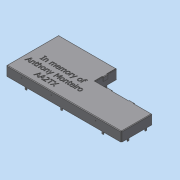
# Autodesk Inventor part: tx_v2_04_cu_shield
Saved by Autodesk Inventor 2014 (Build 180170000, 170)
## iProperties
Created: 2014-03-05
Part Number: tx_v2_04_cu_shield
Material: Generic
Document SubType Name: Sheet Metal
Designer: Robert Davis
Density: 1 g/cm^3
Sheet Metal Rule: Default_mm
Appearance: Default
Flat Pattern Width: 6.62019 cm
Flat Pattern Length: 9.2582 cm
Flat Pattern Area: 61.291 cm^2
Sheet Metal Width: 66.2019 mm
Sheet Metal Length: 92.5820 mm
Sheet Metal Area: 6129.1043 mm^2
Author: Robert Davis
Autodesk Inventor part; units mm, degrees
ref_plane "YZ Plane" through (0, 0, 0) normal (1, 0, 0) x (0, 1, 0)
ref_plane "XZ Plane" through (0, 0, 0) normal (0, 1, 0) x (-1, 0, 0)
ref_plane "XY Plane" through (0, 0, 0) normal (0, 0, 1) x (1, 0, 0)
sketch "Sketch1" plane through (0, 0, 0) normal (0, 0, 1) x (1, 0, 0)
  line L0 (7.5, 46.3001) -> (22.25, 46.3001)
  line L1 (22.25, 46.3001) -> (22.25, 52.2431)
  line L2 (-31.08, 52.2431) -> (-31.08, 45.9911)
  line L3 (-31.08, 45.9911) -> (-37.332, 45.9911)
  line L4 (-37.332, 11.4131) -> (-31.08, 11.4131)
  line L5 (-31.08, 11.4131) -> (-31.08, 5.1611)
  line L6 (45.998, 5.1611) -> (45.998, 11.4131)
  line L7 (45.998, 11.4131) -> (52.25, 11.4131)
  line L8 (52.25, 69.863) -> (46.307, 69.863)
  line L9 (46.307, 69.863) -> (46.307, 31.493)
  line L10 (-17.791, 5.1611) -> (-17.791, 3.6611)
  line L11 (-17.791, 3.6611) -> (-18.791, 3.6611)
  line L12 (-18.791, 3.6611) -> (-18.791, 5.1611)
  line L13 (6.209, 5.1611) -> (6.209, 3.6611)
  line L14 (6.209, 3.6611) -> (5.209, 3.6611)
  line L15 (5.209, 3.6611) -> (5.209, 5.1611)
  line L16 (34.209, 5.1611) -> (34.209, 3.6611)
  line L17 (34.209, 3.6611) -> (33.209, 3.6611)
  line L18 (33.209, 3.6611) -> (33.209, 5.1611)
  line L19 (-31.08, 5.1611) -> (-18.791, 5.1611)
  line L20 (34.209, 5.1611) -> (45.998, 5.1611)
  line L21 (-17.791, 5.1611) -> (5.209, 5.1611)
  line L22 (6.209, 5.1611) -> (33.209, 5.1611)
  line L23 (-37.332, 16.7021) -> (-38.832, 16.7021)
  line L24 (-38.832, 16.7021) -> (-38.832, 17.7021)
  line L25 (-38.832, 17.7021) -> (-37.332, 17.7021)
  line L26 (-37.332, 36.7021) -> (-38.832, 36.7021)
  line L27 (-38.832, 36.7021) -> (-38.832, 37.7021)
  line L28 (-38.832, 37.7021) -> (-37.332, 37.7021)
  line L29 (-18.791, 52.2431) -> (-18.791, 53.7431)
  line L30 (-18.791, 53.7431) -> (-19.791, 53.7431)
  line L31 (-19.791, 53.7431) -> (-19.791, 52.2431)
  line L32 (-3.291, 52.2431) -> (-3.291, 53.7431)
  line L33 (-3.291, 53.7431) -> (-4.291, 53.7431)
  line L34 (-4.291, 53.7431) -> (-4.291, 52.2431)
  line L35 (-4.291, 52.2431) -> (-18.791, 52.2431)
  line L36 (-19.791, 52.2431) -> (-31.08, 52.2431)
  line L37 (-37.332, 45.9911) -> (-37.332, 37.7021)
  line L38 (-37.332, 36.7021) -> (-37.332, 17.7021)
  line L39 (-37.332, 16.7021) -> (-37.332, 11.4131)
  line L40 (15.091, 52.2431) -> (15.091, 53.7431)
  line L41 (15.091, 53.7431) -> (14.091, 53.7431)
  line L42 (14.091, 53.7431) -> (14.091, 52.2431)
  line L43 (52.25, 15.2021) -> (53.75, 15.2021)
  line L44 (53.75, 15.2021) -> (53.75, 16.2021)
  line L45 (53.75, 16.2021) -> (52.25, 16.2021)
  line L46 (52.25, 27.2021) -> (53.75, 27.2021)
  line L47 (53.75, 27.2021) -> (53.75, 28.2021)
  line L48 (53.75, 28.2021) -> (52.25, 28.2021)
  line L49 (52.25, 42.5821) -> (53.75, 42.5821)
  line L50 (53.75, 42.5821) -> (53.75, 43.5821)
  line L51 (53.75, 43.5821) -> (52.25, 43.5821)
  line L52 (52.25, 60.5821) -> (53.75, 60.5821)
  line L53 (53.75, 60.5821) -> (53.75, 61.5821)
  line L54 (53.75, 61.5821) -> (52.25, 61.5821)
  line L55 (22.25, 52.2431) -> (15.091, 52.2431)
  line L56 (14.091, 52.2431) -> (-3.291, 52.2431)
  line L57 (52.25, 61.5821) -> (52.25, 69.863)
  line L58 (52.25, 43.5821) -> (52.25, 60.5821)
  line L59 (52.25, 11.4131) -> (52.25, 15.2021)
  line L60 (52.25, 16.2021) -> (52.25, 27.2021)
  line L61 (52.25, 28.2021) -> (52.25, 42.5821)
  line L62 (7.5, 39.993) -> (10.5, 39.993)
  line L63 (10.5, 39.993) -> (10.5, 36.993)
  line L64 (10.5, 36.993) -> (7.5, 36.993)
  line L65 (31, 31.493) -> (31, 34.493)
  line L66 (31, 34.493) -> (34, 34.493)
  line L67 (34, 34.493) -> (34, 31.493)
  line L68 (16, 31.493) -> (16, 34.493)
  line L69 (16, 34.493) -> (19, 34.493)
  line L70 (19, 34.493) -> (19, 31.493)
  line L71 (7.5, 31.493) -> (7.5, 36.993)
  line L72 (7.5, 39.993) -> (7.5, 46.3001)
  line L73 (34, 31.493) -> (46.307, 31.493)
  line L74 (7.5, 31.493) -> (16, 31.493)
  line L75 (19, 31.493) -> (31, 31.493)
  circle A0 centre (-21.08, 9.1611) radius 0.25
  circle A1 centre (-1.08, 9.1611) radius 0.25
  circle A2 centre (28.92, 9.1611) radius 0.25
  point P0 (0, 0)
  point P1 (-18.291, 3.6611)
  point P2 (5.709, 3.6611)
  point P3 (33.709, 3.6611)
  point P4 (-38.832, 17.2021)
  point P5 (-38.832, 37.2021)
  point P6 (-19.291, 53.7431)
  point P7 (-3.791, 53.7431)
  point P8 (14.591, 53.7431)
  point P9 (53.75, 61.0821)
  point P10 (53.75, 43.0821)
  point P11 (53.75, 27.7021)
  point P12 (53.75, 15.7021)
  point P13 (10.5, 38.493)
  point P14 (17.5, 34.493)
  point P15 (32.5, 34.493)
  dimension "d3" = 14.75
  dimension "d4" = 14.8071
  dimension "d5" = 6.252
  dimension "d7" = 34.578
  dimension "d8" = 77.078
  dimension "d9" = 38.37
  dimension "d10" = 5.943
  dimension "d60" = 5.943
  dimension "d74" = 1.5
  dimension "d75" = 1
  dimension "d76" = 12.789
  dimension "d77" = 24
  dimension "d78" = 28
  dimension "d79" = 5.789
  dimension "d80" = 20
  dimension "d81" = 11.789
  dimension "d82" = 15.5
  dimension "d83" = 4.289
  dimension "d84" = 12
  dimension "d85" = 15.38
  dimension "d86" = 18
  dimension "d87" = 18.382
  dimension "d89" = 38.58
  dimension "d90" = 7.5
  dimension "d91" = 31.493
  dimension "d92" = 3
  dimension "d93" = 3
  dimension "d94" = 7
  dimension "d95" = 10
  dimension "d96" = 15
  dimension "d117" = 0.5
  dimension "d118" = 20
  dimension "d119" = 30
  dimension "d120" = 10
  dimension "d121" = 4
  constraints: 152 end point, 46 equal length, 31 horizontal, 23 vertical, 15 midpoint, 15 parallel, 7 perpendicular, 3 centre point, 2 equal radius
  measures "d3" distance of L0.start L0.end
  measures "d4" distance of L71.start L0.start
  measures "d5" distance of L2.start L2.end
  measures "d7" distance of L3.end L4.start
  measures "d8" distance of L5.end L6.start
  measures "d9" distance of L8.end L9.end
  measures "d10" distance of L0.end L1.end
  measures "d60" distance of L8.start L8.end
  measures "d74" distance of L11.end L12.end
  measures "d75" distance of L10.end L11.end
  measures "d76" distance from line of point (-18.291, 3.661) L5
  measures "d77" distance of point (5.709, 3.661) point (-18.291, 3.661)
  measures "d78" distance of point (33.709, 3.661) point (5.709, 3.661)
  measures "d79" distance from line of point (-38.832, 17.202) L4
  measures "d80" distance of point (-38.832, 37.202) point (-38.832, 17.202)
  measures "d81" distance from line of point (-19.291, 53.743) L2
  measures "d82" distance of point (-3.791, 53.743) point (-19.291, 53.743)
  measures "d83" distance from line of point (53.75, 15.702) L7
  measures "d84" distance of point (53.75, 27.702) point (53.75, 15.702)
  measures "d85" distance of point (53.75, 43.082) point (53.75, 27.702)
  measures "d86" distance of point (53.75, 61.082) point (53.75, 43.082)
  measures "d87" distance of point (14.591, 53.743) point (-3.791, 53.743)
  measures "d89" distance between parallel lines of L2 L72
  measures "d90" distance from line of point (0, 0) L71
  measures "d91" distance from line of point (0, 0) L74
  measures "d92" distance of L62.end L63.end
  measures "d93" distance of L62.start L62.end
  measures "d94" distance from line of point (10.5, 38.493) L74
  measures "d95" distance from line of point (17.5, 34.493) L71
  measures "d96" distance of point (32.5, 34.493) point (17.5, 34.493)
  measures "d117" diameter of A0
  measures "d118" distance of A1.centre A0.centre
  measures "d119" distance of A2.centre A1.centre
  measures "d120" distance from line of A0.centre L5
  measures "d121" distance from line of A0.centre L19
extrude "Plate1" add sketch "Sketch1" along normal blind 0.381
sketch "Sketch4" plane through (0, 0, 0) normal (0, 0, -1) x (-1, 0, 0)
  line L0 (-7.5, 31.493) -> (-7.5, 46.3001) projected
  line L1 (31.08, 52.2431) -> (31.08, 45.9911) projected
  line L2 (31.08, 46.1431) -> (-7.5, 46.1431)
  line L3 (-22.25, 52.2431) -> (31.08, 52.2431) projected
  point P0 (0, 0)
  dimension "d61" = 6.1
  constraints: 2 end point, 2 point on line, 1 horizontal
  measures "d61" distance between parallel lines of L3 L2
fold "Fold2" angle 90 bend radius 0.001 thickness 0.381 k factor 0.44 line from (-31.08, 46.1431, 0) to (7.5, 46.1431, 0) line at bend centre moving side (0, 1, 0) folds toward (0, 0, -1)
sketch "Sketch5" plane through (-31.08, 46.0117, -5.9686) normal (0, -1, 0) x (1, 0, 0)
  line L0 (53.33, 0) -> (0, 0) projected
  line L1 (38.58, 5.943) -> (53.33, 5.943) projected
  line L2 (38.73, 5.943) -> (38.73, 0)
  line L3 (53.33, 5.943) -> (53.33, 0) projected
  point P0 (31.08, 5.9686)
  dimension "d62" = 14.6
  constraints: 2 end point, 2 point on line, 1 vertical
  measures "d62" distance between parallel lines of L2 L3
fold "Fold3" angle 90 bend radius 0.001 thickness 0.381 k factor 0.44 line from (7.65, 46.0117, -0.0256) to (7.65, 46.0117, -5.9686) line at bend centre moving side (1, 0, 0) folds toward (0, -1, 0)
sketch "Sketch6" plane through (0, 0, 0) normal (0, 0, -1) x (-1, 0, 0)
  line L0 (37.332, 11.4131) -> (31.08, 11.4131) projected
  line L1 (31.08, 45.9911) -> (37.332, 45.9911) projected
  line L2 (31.232, 45.9911) -> (31.232, 11.4131)
  line L3 (37.332, 45.9911) -> (37.332, 11.4131) projected
  point P0 (0, 0)
  dimension "d63" = 6.1
  constraints: 2 end point, 2 point on line, 1 vertical
  measures "d63" distance between parallel lines of L3 L2
fold "Fold4" angle 90 bend radius 0.001 thickness 0.381 k factor 0.44 line from (-31.232, 45.9911, 0) to (-31.232, 11.4131, 0) line at bend centre moving side (-1, 0, 0) folds toward (0, 0, -1)
sketch "Sketch7" plane through (0, 0, 0) normal (0, 0, -1) x (-1, 0, 0)
  line L0 (-45.998, 5.1611) -> (-45.998, 11.4131) projected
  line L1 (31.08, 11.4131) -> (31.08, 5.1611) projected
  line L2 (-45.998, 11.2611) -> (31.08, 11.2611)
  line L3 (31.08, 5.1611) -> (-45.998, 5.1611) projected
  point P0 (0, 0)
  dimension "d64" = 6.1
  constraints: 2 end point, 2 point on line, 1 horizontal
  measures "d64" distance between parallel lines of L3 L2
fold "Fold5" angle 90 bend radius 0.001 thickness 0.381 k factor 0.44 line from (45.998, 11.2611, 0) to (-31.08, 11.2611, 0) line at bend centre moving side (0, -1, 0) folds toward (0, 0, -1)
sketch "Sketch8" plane through (0, 0, 0) normal (0, 0, -1) x (-1, 0, 0)
  line L0 (-46.307, 31.493) -> (-7.5, 31.493) projected
  line L1 (-45.998, 11.4131) -> (-52.25, 11.4131) projected
  line L2 (-46.15, 11.4131) -> (-46.15, 31.493)
  line L3 (-52.25, 11.4131) -> (-52.25, 69.863) projected
  point P0 (0, 0)
  dimension "d65" = 6.1
  constraints: 2 end point, 2 point on line, 1 vertical
  measures "d65" distance between parallel lines of L2 L3
fold "Fold6" angle 90 bend radius 0.001 thickness 0.381 k factor 0.44 line from (46.15, 11.4131, 0) to (46.15, 31.493, 0) line at bend centre moving side (1, 0, 0) folds toward (0, 0, -1)
sketch "Sketch9" plane through (46.0186, 11.4131, -5.9686) normal (-1, 0, 0) x (0, 0, 1)
  line L0 (5.943, 58.4499) -> (5.943, 20.0799) projected
  line L1 (0, 0) -> (0, 58.4499) projected
  line L2 (5.943, 20.2299) -> (0, 20.2299)
  line L3 (0, 58.4499) -> (5.943, 58.4499) projected
  point P0 (5.9686, -11.4131)
  dimension "d66" = 38.22
  constraints: 2 end point, 2 point on line, 1 horizontal
  measures "d66" distance between parallel lines of L3 L2
fold "Fold7" angle 90 bend radius 0.001 thickness 0.381 k factor 0.44 line from (46.0186, 31.643, -0.0256) to (46.0186, 31.643, -5.9686) line at bend centre moving side (0, 1, 0) folds toward (-1, 0, 0)
ref_plane "Work Plane1" through (-31.08, 11.202, -5.9686) normal (0, 1, 0) x (1, 0, 0)
ref_plane "Work Plane2" through (-31.2911, 11.4131, -5.9686) normal (1, 0, 0) x (0, 0, -1)
ref_plane "Work Plane3" through (-31.08, 46.2022, -5.9686) normal (0, 1, 0) x (1, 0, 0)
ref_plane "Work Plane4" through (46.2091, 11.4131, -5.9686) normal (1, 0, 0) x (0, 0, -1)
ref_plane "Work Plane5" through (7.7091, 31.5431, -5.9686) normal (1, 0, 0) x (0, 0, -1)
ref_plane "Work Plane6" through (7.93, 31.7021, -5.9686) normal (0, -1, 0) x (1, 0, 0)
ref_plane "Work Plane7" through (-18.291, 11.0115, -7.4686) normal (-1, 0, 0) x (0, 0, 1)
ref_plane "Work Plane8" through (5.709, 11.0115, -7.4686) normal (-1, 0, 0) x (0, 0, 1)
ref_plane "Work Plane9" through (33.709, 11.0115, -7.4686) normal (-1, 0, 0) x (0, 0, 1)
ref_plane "Work Plane10" through (46.3996, 15.7021, -7.4686) normal (0, -1, 0) x (1, 0, 0)
ref_plane "Work Plane11" through (46.3996, 27.7021, -7.4686) normal (0, -1, 0) x (1, 0, 0)
ref_plane "Work Plane12" through (34.7109, 31.8926, -7.4686) normal (1, 0, 0) x (0, 0, -1)
ref_plane "Work Plane13" through (16.7109, 31.8926, -7.4686) normal (1, 0, 0) x (0, 0, -1)
ref_plane "Work Plane14" through (7.8996, 39.2021, -7.4686) normal (0, 1, 0) x (1, 0, 0)
ref_plane "Work Plane15" through (-3.791, 46.3927, -7.4686) normal (-1, 0, 0) x (0, 0, 1)
ref_plane "Work Plane16" through (-19.291, 46.3927, -7.4686) normal (-1, 0, 0) x (0, 0, 1)
ref_plane "Work Plane17" through (-31.4816, 37.2021, -7.4686) normal (0, 1, 0) x (1, 0, 0)
ref_plane "Work Plane18" through (-31.4816, 17.2021, -7.4686) normal (0, 1, 0) x (1, 0, 0)
sketch "Sketch11" plane through (0, 0, 0) normal (0, 0, -1) x (-1, 0, 0)
  line L0 (-10.5, 39.993) -> (-7.5, 39.993) projected
  line L1 (-10.5, 36.993) -> (-10.5, 39.993) projected
  line L2 (-7.5, 36.993) -> (-10.5, 36.993) projected
  line L3 (-8.032, 36.993) -> (-8.032, 39.993)
  point P0 (0, 0)
  dimension "d97" = 2.468
  constraints: 2 end point, 2 point on line, 1 vertical
  measures "d97" distance between parallel lines of L3 L1
fold "Fold8" angle 90 bend radius 0.001 thickness 0.381 k factor 0.44 line from (8.032, 36.993, 0) to (8.032, 39.993, 0) line at bend centre moving side (1, 0, 0) folds toward (0, 0, -1)
sketch "Sketch12" plane through (0, 0, 0) normal (0, 0, -1) x (-1, 0, 0)
  line L0 (-16, 34.493) -> (-16, 31.493) projected
  line L1 (-34, 34.493) -> (-31, 34.493) projected
  line L2 (-34, 31.493) -> (-34, 34.493) projected
  line L3 (-16, 32.025) -> (-34, 32.025)
  point P0 (0, 0)
  dimension "d104" = 2.468
  constraints: 2 end point, 2 point on line, 1 horizontal
  measures "d104" distance between parallel lines of L3 L1
fold "Fold10" angle 90 bend radius 0.001 thickness 0.381 k factor 0.44 line from (16, 32.025, 0) to (34, 32.025, 0) line at bend centre moving side (0, 1, 0) folds toward (0, 0, -1)
sketch "Sketch13" plane through (0, 0, 0.381) normal (0, 0, 1) x (1, 0, 0)
  line L0 (-28.539, 29.8177) -> (9.1186, 29.8177) construction
  line L1 (9.1186, 29.8177) -> (9.1186, 14.6137) construction
  line L2 (9.1186, 14.6137) -> (-28.539, 14.6137) construction
  line L3 (-28.539, 14.6137) -> (-28.539, 29.8177) construction
  line L4 (-22.682, 26.139) -> (-24.0378, 26.139)
  line L5 (-24.0378, 26.139) -> (-24.0378, 26.4964)
  line L6 (-24.0378, 26.4964) -> (-23.5925, 26.4964)
  line L7 (-23.5925, 26.4964) -> (-23.5925, 29.2816)
  line L8 (-23.5925, 29.2816) -> (-24.0378, 29.2816)
  line L9 (-24.0378, 29.2816) -> (-24.0378, 29.639)
  line L10 (-24.0378, 29.639) -> (-22.682, 29.639)
  line L11 (-22.682, 29.639) -> (-22.682, 29.2816)
  line L12 (-22.682, 29.2816) -> (-23.1273, 29.2816)
  line L13 (-23.1273, 29.2816) -> (-23.1273, 26.4964)
  line L14 (-23.1273, 26.4964) -> (-22.682, 26.4964)
  line L15 (-22.682, 26.4964) -> (-22.682, 26.139)
  line L16 (-20.0783, 26.139) -> (-20.5207, 26.139)
  line L17 (-20.5207, 26.139) -> (-20.5207, 27.6366)
  spline S0 degree 2 poles (-20.5207, 27.6366) (-20.5207, 27.8181) (-20.5548, 28.1301) (-20.6058, 28.2237) knots 0 0 0 1 2 2 2
  spline S1 degree 2 poles (-20.6058, 28.2237) (-20.6597, 28.323) (-20.8526, 28.4194) (-21.0171, 28.4194) knots 0 0 0 1 2 2 2
  spline S2 degree 2 poles (-21.0171, 28.4194) (-21.1816, 28.4194) (-21.5305, 28.2435) (-21.6978, 28.1017) knots 0 0 0 1 2 2 2
  line L18 (-21.6978, 28.1017) -> (-21.6978, 26.139)
  line L19 (-21.6978, 26.139) -> (-22.1403, 26.139)
  line L20 (-22.1403, 26.139) -> (-22.1403, 28.7654)
  line L21 (-22.1403, 28.7654) -> (-21.6978, 28.7654)
  line L22 (-21.6978, 28.7654) -> (-21.6978, 28.4733)
  spline S3 degree 2 poles (-21.6978, 28.4733) (-21.4993, 28.652) (-21.1164, 28.8392) (-20.9008, 28.8392) knots 0 0 0 1 2 2 2
  spline S4 degree 2 poles (-20.9008, 28.8392) (-20.5151, 28.8392) (-20.0783, 28.3286) (-20.0783, 27.8436) knots 0 0 0 1 2 2 2
  line L23 (-20.0783, 27.8436) -> (-20.0783, 26.139)
  line L24 (-14.9758, 26.139) -> (-14.9758, 27.6593)
  spline S5 degree 2 poles (-14.9758, 27.6593) (-14.9758, 27.8408) (-15.0041, 28.1499) (-15.0495, 28.235) knots 0 0 0 1 2 2 2
  spline S6 degree 2 poles (-15.0495, 28.235) (-15.0949, 28.3286) (-15.2679, 28.4194) (-15.4182, 28.4194) knots 0 0 0 1 2 2 2
  spline S7 degree 2 poles (-15.4182, 28.4194) (-15.5544, 28.4194) (-15.8664, 28.2521) (-16.0309, 28.0932) knots 0 0 0 1 2 2 2
  spline S8 degree 2 poles (-16.0309, 28.0932) (-16.028, 28.0535) (-16.0224, 27.9429) (-16.0224, 27.8692) knots 0 0 0 1 2 2 2
  line L25 (-16.0224, 27.8692) -> (-16.0224, 26.139)
  line L26 (-16.0224, 26.139) -> (-16.4648, 26.139)
  line L27 (-16.4648, 26.139) -> (-16.4648, 27.6593)
  spline S9 degree 2 poles (-16.4648, 27.6593) (-16.4648, 27.8408) (-16.4932, 28.1499) (-16.5386, 28.235) knots 0 0 0 1 2 2 2
  spline S10 degree 2 poles (-16.5386, 28.235) (-16.584, 28.3286) (-16.757, 28.4194) (-16.9073, 28.4194) knots 0 0 0 1 2 2 2
  spline S11 degree 2 poles (-16.9073, 28.4194) (-17.0491, 28.4194) (-17.3639, 28.2407) (-17.5114, 28.1017) knots 0 0 0 1 2 2 2
  line L28 (-17.5114, 28.1017) -> (-17.5114, 26.139)
  line L29 (-17.5114, 26.139) -> (-17.9539, 26.139)
  line L30 (-17.9539, 26.139) -> (-17.9539, 28.7654)
  line L31 (-17.9539, 28.7654) -> (-17.5114, 28.7654)
  line L32 (-17.5114, 28.7654) -> (-17.5114, 28.4761)
  spline S12 degree 2 poles (-17.5114, 28.4761) (-17.3384, 28.6491) (-16.9981, 28.8392) (-16.7938, 28.8392) knots 0 0 0 1 2 2 2
  spline S13 degree 2 poles (-16.7938, 28.8392) (-16.5613, 28.8392) (-16.201, 28.6264) (-16.1075, 28.3854) knots 0 0 0 1 2 2 2
  spline S14 degree 2 poles (-16.1075, 28.3854) (-15.9061, 28.6094) (-15.526, 28.8392) (-15.3048, 28.8392) knots 0 0 0 1 2 2 2
  spline S15 degree 2 poles (-15.3048, 28.8392) (-15.1346, 28.8392) (-14.8566, 28.7342) (-14.7545, 28.6151) knots 0 0 0 1 2 2 2
  spline S16 degree 2 poles (-14.7545, 28.6151) (-14.6496, 28.496) (-14.5333, 28.1386) (-14.5333, 27.8692) knots 0 0 0 1 2 2 2
  line L33 (-14.5333, 27.8692) -> (-14.5333, 26.139)
  line L34 (-14.5333, 26.139) -> (-14.9758, 26.139)
  spline S17 degree 2 poles (-12.772, 26.0794) (-13.4016, 26.0794) (-14.0937, 26.7857) (-14.0937, 27.438) knots 0 0 0 1 2 2 2
  spline S18 degree 2 poles (-14.0937, 27.438) (-14.0937, 28.079) (-13.4215, 28.8392) (-12.8797, 28.8392) knots 0 0 0 1 2 2 2
  spline S19 degree 2 poles (-12.8797, 28.8392) (-12.6358, 28.8392) (-12.2586, 28.6974) (-12.1196, 28.547) knots 0 0 0 1 2 2 2
  spline S20 degree 2 poles (-12.1196, 28.547) (-11.9778, 28.3967) (-11.8275, 27.9627) (-11.8275, 27.6479) knots 0 0 0 1 2 2 2
  line L35 (-11.8275, 27.6479) -> (-11.8275, 27.4068)
  line L36 (-11.8275, 27.4068) -> (-13.6455, 27.4068)
  spline S21 degree 2 poles (-13.6455, 27.4068) (-13.6455, 26.9502) (-13.1861, 26.4652) (-12.7776, 26.4652) knots 0 0 0 1 2 2 2
  spline S22 degree 2 poles (-12.7776, 26.4652) (-12.633, 26.4652) (-12.3522, 26.5304) (-12.2387, 26.5815) knots 0 0 0 1 2 2 2
  spline S23 degree 2 poles (-12.2387, 26.5815) (-12.1196, 26.6382) (-11.9551, 26.7375) (-11.9012, 26.7828) knots 0 0 0 1 2 2 2
  line L37 (-11.9012, 26.7828) -> (-11.8757, 26.7828)
  line L38 (-11.8757, 26.7828) -> (-11.8757, 26.3007)
  spline S24 degree 2 poles (-11.8757, 26.3007) (-11.9523, 26.2695) (-12.1848, 26.1787) (-12.2756, 26.1532) knots 0 0 0 1 2 2 2
  spline S25 degree 2 poles (-12.2756, 26.1532) (-12.4032, 26.1163) (-12.6131, 26.0794) (-12.772, 26.0794) knots 0 0 0 1 2 2 2
  spline S26 degree 2 poles (-12.2586, 27.7444) (-12.2643, 27.923) (-12.338, 28.184) (-12.4089, 28.2719) knots 0 0 0 1 2 2 2
  spline S27 degree 2 poles (-12.4089, 28.2719) (-12.4855, 28.3712) (-12.7266, 28.4761) (-12.9053, 28.4761) knots 0 0 0 1 2 2 2
  spline S28 degree 2 poles (-12.9053, 28.4761) (-13.0811, 28.4761) (-13.3279, 28.3712) (-13.43, 28.2691) knots 0 0 0 1 2 2 2
  spline S29 degree 2 poles (-13.43, 28.2691) (-13.5293, 28.1641) (-13.6314, 27.9117) (-13.6455, 27.7444) knots 0 0 0 1 2 2 2
  line L39 (-13.6455, 27.7444) -> (-12.2586, 27.7444)
  line L40 (-8.4012, 26.139) -> (-8.4012, 27.6593)
  spline S30 degree 2 poles (-8.4012, 27.6593) (-8.4012, 27.8408) (-8.4296, 28.1499) (-8.475, 28.235) knots 0 0 0 1 2 2 2
  spline S31 degree 2 poles (-8.475, 28.235) (-8.5203, 28.3286) (-8.6934, 28.4194) (-8.8437, 28.4194) knots 0 0 0 1 2 2 2
  spline S32 degree 2 poles (-8.8437, 28.4194) (-8.9798, 28.4194) (-9.2918, 28.2521) (-9.4563, 28.0932) knots 0 0 0 1 2 2 2
  spline S33 degree 2 poles (-9.4563, 28.0932) (-9.4535, 28.0535) (-9.4478, 27.9429) (-9.4478, 27.8692) knots 0 0 0 1 2 2 2
  line L41 (-9.4478, 27.8692) -> (-9.4478, 26.139)
  line L42 (-9.4478, 26.139) -> (-9.8903, 26.139)
  line L43 (-9.8903, 26.139) -> (-9.8903, 27.6593)
  spline S34 degree 2 poles (-9.8903, 27.6593) (-9.8903, 27.8408) (-9.9186, 28.1499) (-9.964, 28.235) knots 0 0 0 1 2 2 2
  spline S35 degree 2 poles (-9.964, 28.235) (-10.0094, 28.3286) (-10.1824, 28.4194) (-10.3327, 28.4194) knots 0 0 0 1 2 2 2
  spline S36 degree 2 poles (-10.3327, 28.4194) (-10.4746, 28.4194) (-10.7894, 28.2407) (-10.9369, 28.1017) knots 0 0 0 1 2 2 2
  line L44 (-10.9369, 28.1017) -> (-10.9369, 26.139)
  line L45 (-10.9369, 26.139) -> (-11.3793, 26.139)
  line L46 (-11.3793, 26.139) -> (-11.3793, 28.7654)
  line L47 (-11.3793, 28.7654) -> (-10.9369, 28.7654)
  line L48 (-10.9369, 28.7654) -> (-10.9369, 28.4761)
  spline S37 degree 2 poles (-10.9369, 28.4761) (-10.7639, 28.6491) (-10.4235, 28.8392) (-10.2193, 28.8392) knots 0 0 0 1 2 2 2
  spline S38 degree 2 poles (-10.2193, 28.8392) (-9.9867, 28.8392) (-9.6265, 28.6264) (-9.5329, 28.3854) knots 0 0 0 1 2 2 2
  spline S39 degree 2 poles (-9.5329, 28.3854) (-9.3315, 28.6094) (-8.9515, 28.8392) (-8.7302, 28.8392) knots 0 0 0 1 2 2 2
  spline S40 degree 2 poles (-8.7302, 28.8392) (-8.56, 28.8392) (-8.2821, 28.7342) (-8.18, 28.6151) knots 0 0 0 1 2 2 2
  spline S41 degree 2 poles (-8.18, 28.6151) (-8.075, 28.496) (-7.9587, 28.1386) (-7.9587, 27.8692) knots 0 0 0 1 2 2 2
  line L49 (-7.9587, 27.8692) -> (-7.9587, 26.139)
  line L50 (-7.9587, 26.139) -> (-8.4012, 26.139)
  spline S42 degree 2 poles (-5.1792, 27.4522) (-5.1792, 26.7885) (-5.8173, 26.0653) (-6.3506, 26.0653) knots 0 0 0 1 2 2 2
  spline S43 degree 2 poles (-6.3506, 26.0653) (-6.898, 26.0653) (-7.5248, 26.8112) (-7.5248, 27.4522) knots 0 0 0 1 2 2 2
  spline S44 degree 2 poles (-7.5248, 27.4522) (-7.5248, 28.1102) (-6.8781, 28.8392) (-6.3506, 28.8392) knots 0 0 0 1 2 2 2
  spline S45 degree 2 poles (-6.3506, 28.8392) (-5.8173, 28.8392) (-5.1792, 28.1131) (-5.1792, 27.4522) knots 0 0 0 1 2 2 2
  spline S46 degree 2 poles (-5.6358, 27.4522) (-5.6358, 27.9627) (-6.0074, 28.4591) (-6.3506, 28.4591) knots 0 0 0 1 2 2 2
  spline S47 degree 2 poles (-6.3506, 28.4591) (-6.6938, 28.4591) (-7.0681, 27.9627) (-7.0681, 27.4522) knots 0 0 0 1 2 2 2
  spline S48 degree 2 poles (-7.0681, 27.4522) (-7.0681, 26.9559) (-6.6938, 26.4453) (-6.3506, 26.4453) knots 0 0 0 1 2 2 2
  spline S49 degree 2 poles (-6.3506, 26.4453) (-6.0102, 26.4453) (-5.6358, 26.9474) (-5.6358, 27.4522) knots 0 0 0 1 2 2 2
  line L51 (-3.3327, 28.2918) -> (-3.3554, 28.2918)
  spline S50 degree 2 poles (-3.3554, 28.2918) (-3.4065, 28.3059) (-3.5171, 28.3116) (-3.5937, 28.3116) knots 0 0 0 1 2 2 2
  spline S51 degree 2 poles (-3.5937, 28.3116) (-3.7724, 28.3116) (-4.1241, 28.1556) (-4.2829, 28.0025) knots 0 0 0 1 2 2 2
  line L52 (-4.2829, 28.0025) -> (-4.2829, 26.139)
  line L53 (-4.2829, 26.139) -> (-4.7254, 26.139)
  line L54 (-4.7254, 26.139) -> (-4.7254, 28.7654)
  line L55 (-4.7254, 28.7654) -> (-4.2829, 28.7654)
  line L56 (-4.2829, 28.7654) -> (-4.2829, 28.374)
  spline S52 degree 2 poles (-4.2829, 28.374) (-4.0418, 28.5896) (-3.6816, 28.7654) (-3.5114, 28.7654) knots 0 0 0 1 2 2 2
  spline S53 degree 2 poles (-3.5114, 28.7654) (-3.4434, 28.7654) (-3.3753, 28.7597) (-3.3327, 28.7512) knots 0 0 0 1 2 2 2
  line L57 (-3.3327, 28.7512) -> (-3.3327, 28.2918)
  line L58 (-0.9275, 28.7654) -> (-2.34, 25.1718)
  line L59 (-2.34, 25.1718) -> (-2.8137, 25.1718)
  line L60 (-2.8137, 25.1718) -> (-2.3429, 26.2666)
  line L61 (-2.3429, 26.2666) -> (-3.2959, 28.7654)
  line L62 (-3.2959, 28.7654) -> (-2.8194, 28.7654)
  line L63 (-2.8194, 28.7654) -> (-2.1018, 26.8197)
  line L64 (-2.1018, 26.8197) -> (-1.387, 28.7654)
  line L65 (-1.387, 28.7654) -> (-0.9275, 28.7654)
  spline S54 degree 2 poles (3.0688, 27.4522) (3.0688, 26.7885) (2.4306, 26.0653) (1.8974, 26.0653) knots 0 0 0 1 2 2 2
  spline S55 degree 2 poles (1.8974, 26.0653) (1.35, 26.0653) (0.7232, 26.8112) (0.7232, 27.4522) knots 0 0 0 1 2 2 2
  spline S56 degree 2 poles (0.7232, 27.4522) (0.7232, 28.1102) (1.3699, 28.8392) (1.8974, 28.8392) knots 0 0 0 1 2 2 2
  spline S57 degree 2 poles (1.8974, 28.8392) (2.4306, 28.8392) (3.0688, 28.1131) (3.0688, 27.4522) knots 0 0 0 1 2 2 2
  spline S58 degree 2 poles (2.6122, 27.4522) (2.6122, 27.9627) (2.2406, 28.4591) (1.8974, 28.4591) knots 0 0 0 1 2 2 2
  spline S59 degree 2 poles (1.8974, 28.4591) (1.5542, 28.4591) (1.1798, 27.9627) (1.1798, 27.4522) knots 0 0 0 1 2 2 2
  spline S60 degree 2 poles (1.1798, 27.4522) (1.1798, 26.9559) (1.5542, 26.4453) (1.8974, 26.4453) knots 0 0 0 1 2 2 2
  spline S61 degree 2 poles (1.8974, 26.4453) (2.2378, 26.4453) (2.6122, 26.9474) (2.6122, 27.4522) knots 0 0 0 1 2 2 2
  line L66 (4.9039, 29.3696) -> (4.8812, 29.3696)
  spline S62 degree 2 poles (4.8812, 29.3696) (4.8216, 29.3922) (4.6004, 29.432) (4.5125, 29.432) knots 0 0 0 1 2 2 2
  spline S63 degree 2 poles (4.5125, 29.432) (4.2345, 29.432) (3.9963, 29.1824) (3.9963, 28.8533) knots 0 0 0 1 2 2 2
  line L67 (3.9963, 28.8533) -> (3.9963, 28.7654)
  line L68 (3.9963, 28.7654) -> (4.728, 28.7654)
  line L69 (4.728, 28.7654) -> (4.728, 28.3995)
  line L70 (4.728, 28.3995) -> (4.0105, 28.3995)
  line L71 (4.0105, 28.3995) -> (4.0105, 26.139)
  line L72 (4.0105, 26.139) -> (3.568, 26.139)
  line L73 (3.568, 26.139) -> (3.568, 28.3995)
  line L74 (3.568, 28.3995) -> (3.2702, 28.3995)
  line L75 (3.2702, 28.3995) -> (3.2702, 28.7654)
  line L76 (3.2702, 28.7654) -> (3.568, 28.7654)
  line L77 (3.568, 28.7654) -> (3.568, 28.8533)
  spline S64 degree 2 poles (3.568, 28.8533) (3.568, 29.3242) (4.0246, 29.8177) (4.4501, 29.8177) knots 0 0 0 1 2 2 2
  spline S65 degree 2 poles (4.4501, 29.8177) (4.572, 29.8177) (4.8075, 29.7922) (4.9039, 29.7751) knots 0 0 0 1 2 2 2
  line L78 (4.9039, 29.7751) -> (4.9039, 29.3696)
  line L79 (-28.5617, 20.3763) -> (-27.3818, 23.8763)
  line L80 (-27.3818, 23.8763) -> (-26.8088, 23.8763)
  line L81 (-26.8088, 23.8763) -> (-25.6289, 20.3763)
  line L82 (-25.6289, 20.3763) -> (-26.1196, 20.3763)
  line L83 (-26.1196, 20.3763) -> (-26.4373, 21.3549)
  line L84 (-26.4373, 21.3549) -> (-27.7732, 21.3549)
  line L85 (-27.7732, 21.3549) -> (-28.0908, 20.3763)
  line L86 (-28.0908, 20.3763) -> (-28.5617, 20.3763)
  line L87 (-26.5649, 21.752) -> (-27.1066, 23.3998)
  line L88 (-27.1066, 23.3998) -> (-27.6455, 21.752)
  line L89 (-27.6455, 21.752) -> (-26.5649, 21.752)
  line L90 (-23.2691, 20.3763) -> (-23.7116, 20.3763)
  line L91 (-23.7116, 20.3763) -> (-23.7116, 21.8739)
  spline S66 degree 2 poles (-23.7116, 21.8739) (-23.7116, 22.0554) (-23.7456, 22.3674) (-23.7967, 22.461) knots 0 0 0 1 2 2 2
  spline S67 degree 2 poles (-23.7967, 22.461) (-23.8506, 22.5603) (-24.0434, 22.6567) (-24.2079, 22.6567) knots 0 0 0 1 2 2 2
  spline S68 degree 2 poles (-24.2079, 22.6567) (-24.3724, 22.6567) (-24.7213, 22.4809) (-24.8887, 22.3391) knots 0 0 0 1 2 2 2
  line L92 (-24.8887, 22.3391) -> (-24.8887, 20.3763)
  line L93 (-24.8887, 20.3763) -> (-25.3311, 20.3763)
  line L94 (-25.3311, 20.3763) -> (-25.3311, 23.0028)
  line L95 (-25.3311, 23.0028) -> (-24.8887, 23.0028)
  line L96 (-24.8887, 23.0028) -> (-24.8887, 22.7106)
  spline S69 degree 2 poles (-24.8887, 22.7106) (-24.6901, 22.8893) (-24.3072, 23.0765) (-24.0916, 23.0765) knots 0 0 0 1 2 2 2
  spline S70 degree 2 poles (-24.0916, 23.0765) (-23.7059, 23.0765) (-23.2691, 22.566) (-23.2691, 22.081) knots 0 0 0 1 2 2 2
  line L97 (-23.2691, 22.081) -> (-23.2691, 20.3763)
  spline S71 degree 2 poles (-21.8538, 20.3253) (-22.214, 20.3253) (-22.6196, 20.7366) (-22.6196, 21.1819) knots 0 0 0 1 2 2 2
  line L98 (-22.6196, 21.1819) -> (-22.6196, 22.6369)
  line L99 (-22.6196, 22.6369) -> (-22.9174, 22.6369)
  line L100 (-22.9174, 22.6369) -> (-22.9174, 23.0028)
  line L101 (-22.9174, 23.0028) -> (-22.6196, 23.0028)
  line L102 (-22.6196, 23.0028) -> (-22.6196, 23.7572)
  line L103 (-22.6196, 23.7572) -> (-22.1771, 23.7572)
  line L104 (-22.1771, 23.7572) -> (-22.1771, 23.0028)
  line L105 (-22.1771, 23.0028) -> (-21.3631, 23.0028)
  line L106 (-21.3631, 23.0028) -> (-21.3631, 22.6369)
  line L107 (-21.3631, 22.6369) -> (-22.1771, 22.6369)
  line L108 (-22.1771, 22.6369) -> (-22.1771, 21.3861)
  spline S72 degree 2 poles (-22.1771, 21.3861) (-22.1771, 21.1875) (-22.163, 20.9691) (-22.1147, 20.8755) knots 0 0 0 1 2 2 2
  spline S73 degree 2 poles (-22.1147, 20.8755) (-22.075, 20.7933) (-21.8963, 20.711) (-21.7432, 20.711) knots 0 0 0 1 2 2 2
  spline S74 degree 2 poles (-21.7432, 20.711) (-21.6354, 20.711) (-21.434, 20.7763) (-21.3887, 20.7961) knots 0 0 0 1 2 2 2
  line L109 (-21.3887, 20.7961) -> (-21.3631, 20.7961)
  line L110 (-21.3631, 20.7961) -> (-21.3631, 20.399)
  spline S75 degree 2 poles (-21.3631, 20.399) (-21.4879, 20.365) (-21.7432, 20.3253) (-21.8538, 20.3253) knots 0 0 0 1 2 2 2
  line L111 (-18.975, 20.3763) -> (-19.4174, 20.3763)
  line L112 (-19.4174, 20.3763) -> (-19.4174, 21.8739)
  spline S76 degree 2 poles (-19.4174, 21.8739) (-19.4174, 22.0554) (-19.4515, 22.3674) (-19.5025, 22.461) knots 0 0 0 1 2 2 2
  spline S77 degree 2 poles (-19.5025, 22.461) (-19.5564, 22.5603) (-19.7493, 22.6567) (-19.9138, 22.6567) knots 0 0 0 1 2 2 2
  spline S78 degree 2 poles (-19.9138, 22.6567) (-20.0783, 22.6567) (-20.4271, 22.4809) (-20.5945, 22.3391) knots 0 0 0 1 2 2 2
  line L113 (-20.5945, 22.3391) -> (-20.5945, 20.3763)
  line L114 (-20.5945, 20.3763) -> (-21.0369, 20.3763)
  line L115 (-21.0369, 20.3763) -> (-21.0369, 24.0323)
  line L116 (-21.0369, 24.0323) -> (-20.5945, 24.0323)
  line L117 (-20.5945, 24.0323) -> (-20.5945, 22.7106)
  spline S79 degree 2 poles (-20.5945, 22.7106) (-20.3959, 22.8893) (-20.013, 23.0765) (-19.7975, 23.0765) knots 0 0 0 1 2 2 2
  spline S80 degree 2 poles (-19.7975, 23.0765) (-19.4117, 23.0765) (-18.975, 22.566) (-18.975, 22.081) knots 0 0 0 1 2 2 2
  line L118 (-18.975, 22.081) -> (-18.975, 20.3763)
  spline S81 degree 2 poles (-16.1954, 21.6896) (-16.1954, 21.0259) (-16.8335, 20.3026) (-17.3668, 20.3026) knots 0 0 0 1 2 2 2
  spline S82 degree 2 poles (-17.3668, 20.3026) (-17.9142, 20.3026) (-18.541, 21.0486) (-18.541, 21.6896) knots 0 0 0 1 2 2 2
  spline S83 degree 2 poles (-18.541, 21.6896) (-18.541, 22.3476) (-17.8943, 23.0765) (-17.3668, 23.0765) knots 0 0 0 1 2 2 2
  spline S84 degree 2 poles (-17.3668, 23.0765) (-16.8335, 23.0765) (-16.1954, 22.3504) (-16.1954, 21.6896) knots 0 0 0 1 2 2 2
  spline S85 degree 2 poles (-16.652, 21.6896) (-16.652, 22.2001) (-17.0236, 22.6964) (-17.3668, 22.6964) knots 0 0 0 1 2 2 2
  spline S86 degree 2 poles (-17.3668, 22.6964) (-17.71, 22.6964) (-18.0844, 22.2001) (-18.0844, 21.6896) knots 0 0 0 1 2 2 2
  spline S87 degree 2 poles (-18.0844, 21.6896) (-18.0844, 21.1932) (-17.71, 20.6827) (-17.3668, 20.6827) knots 0 0 0 1 2 2 2
  spline S88 degree 2 poles (-17.3668, 20.6827) (-17.0264, 20.6827) (-16.652, 21.1847) (-16.652, 21.6896) knots 0 0 0 1 2 2 2
  line L119 (-13.6796, 20.3763) -> (-14.122, 20.3763)
  line L120 (-14.122, 20.3763) -> (-14.122, 21.8739)
  spline S89 degree 2 poles (-14.122, 21.8739) (-14.122, 22.0554) (-14.1561, 22.3674) (-14.2071, 22.461) knots 0 0 0 1 2 2 2
  spline S90 degree 2 poles (-14.2071, 22.461) (-14.261, 22.5603) (-14.4539, 22.6567) (-14.6184, 22.6567) knots 0 0 0 1 2 2 2
  spline S91 degree 2 poles (-14.6184, 22.6567) (-14.7829, 22.6567) (-15.1318, 22.4809) (-15.2991, 22.3391) knots 0 0 0 1 2 2 2
  line L121 (-15.2991, 22.3391) -> (-15.2991, 20.3763)
  line L122 (-15.2991, 20.3763) -> (-15.7416, 20.3763)
  line L123 (-15.7416, 20.3763) -> (-15.7416, 23.0028)
  line L124 (-15.7416, 23.0028) -> (-15.2991, 23.0028)
  line L125 (-15.2991, 23.0028) -> (-15.2991, 22.7106)
  spline S92 degree 2 poles (-15.2991, 22.7106) (-15.1006, 22.8893) (-14.7177, 23.0765) (-14.5021, 23.0765) knots 0 0 0 1 2 2 2
  spline S93 degree 2 poles (-14.5021, 23.0765) (-14.1164, 23.0765) (-13.6796, 22.566) (-13.6796, 22.081) knots 0 0 0 1 2 2 2
  line L126 (-13.6796, 22.081) -> (-13.6796, 20.3763)
  line L127 (-10.9964, 23.0028) -> (-12.4089, 19.4092)
  line L128 (-12.4089, 19.4092) -> (-12.8826, 19.4092)
  line L129 (-12.8826, 19.4092) -> (-12.4117, 20.504)
  line L130 (-12.4117, 20.504) -> (-13.3647, 23.0028)
  line L131 (-13.3647, 23.0028) -> (-12.8882, 23.0028)
  line L132 (-12.8882, 23.0028) -> (-12.1707, 21.0571)
  line L133 (-12.1707, 21.0571) -> (-11.4559, 23.0028)
  line L134 (-11.4559, 23.0028) -> (-10.9964, 23.0028)
  line L135 (-6.1237, 20.3763) -> (-6.5888, 20.3763)
  line L136 (-6.5888, 20.3763) -> (-6.5888, 23.3913)
  line L137 (-6.5888, 23.3913) -> (-7.5021, 21.3407)
  line L138 (-7.5021, 21.3407) -> (-7.7857, 21.3407)
  line L139 (-7.7857, 21.3407) -> (-8.6905, 23.3913)
  line L140 (-8.6905, 23.3913) -> (-8.6905, 20.3763)
  line L141 (-8.6905, 20.3763) -> (-9.1245, 20.3763)
  line L142 (-9.1245, 20.3763) -> (-9.1245, 23.8763)
  line L143 (-9.1245, 23.8763) -> (-8.4891, 23.8763)
  line L144 (-8.4891, 23.8763) -> (-7.6156, 21.9278)
  line L145 (-7.6156, 21.9278) -> (-6.7703, 23.8763)
  line L146 (-6.7703, 23.8763) -> (-6.1237, 23.8763)
  line L147 (-6.1237, 23.8763) -> (-6.1237, 20.3763)
  spline S94 degree 2 poles (-3.2902, 21.6896) (-3.2902, 21.0259) (-3.9284, 20.3026) (-4.4616, 20.3026) knots 0 0 0 1 2 2 2
  spline S95 degree 2 poles (-4.4616, 20.3026) (-5.009, 20.3026) (-5.6358, 21.0486) (-5.6358, 21.6896) knots 0 0 0 1 2 2 2
  spline S96 degree 2 poles (-5.6358, 21.6896) (-5.6358, 22.3476) (-4.9891, 23.0765) (-4.4616, 23.0765) knots 0 0 0 1 2 2 2
  spline S97 degree 2 poles (-4.4616, 23.0765) (-3.9284, 23.0765) (-3.2902, 22.3504) (-3.2902, 21.6896) knots 0 0 0 1 2 2 2
  spline S98 degree 2 poles (-3.7468, 21.6896) (-3.7468, 22.2001) (-4.1184, 22.6964) (-4.4616, 22.6964) knots 0 0 0 1 2 2 2
  spline S99 degree 2 poles (-4.4616, 22.6964) (-4.8048, 22.6964) (-5.1792, 22.2001) (-5.1792, 21.6896) knots 0 0 0 1 2 2 2
  spline S100 degree 2 poles (-5.1792, 21.6896) (-5.1792, 21.1932) (-4.8048, 20.6827) (-4.4616, 20.6827) knots 0 0 0 1 2 2 2
  spline S101 degree 2 poles (-4.4616, 20.6827) (-4.1212, 20.6827) (-3.7468, 21.1847) (-3.7468, 21.6896) knots 0 0 0 1 2 2 2
  line L148 (-0.7744, 20.3763) -> (-1.2169, 20.3763)
  line L149 (-1.2169, 20.3763) -> (-1.2169, 21.8739)
  spline S102 degree 2 poles (-1.2169, 21.8739) (-1.2169, 22.0554) (-1.2509, 22.3674) (-1.3019, 22.461) knots 0 0 0 1 2 2 2
  spline S103 degree 2 poles (-1.3019, 22.461) (-1.3558, 22.5603) (-1.5487, 22.6567) (-1.7132, 22.6567) knots 0 0 0 1 2 2 2
  spline S104 degree 2 poles (-1.7132, 22.6567) (-1.8777, 22.6567) (-2.2266, 22.4809) (-2.3939, 22.3391) knots 0 0 0 1 2 2 2
  line L150 (-2.3939, 22.3391) -> (-2.3939, 20.3763)
  line L151 (-2.3939, 20.3763) -> (-2.8364, 20.3763)
  line L152 (-2.8364, 20.3763) -> (-2.8364, 23.0028)
  line L153 (-2.8364, 23.0028) -> (-2.3939, 23.0028)
  line L154 (-2.3939, 23.0028) -> (-2.3939, 22.7106)
  spline S105 degree 2 poles (-2.3939, 22.7106) (-2.1954, 22.8893) (-1.8125, 23.0765) (-1.5969, 23.0765) knots 0 0 0 1 2 2 2
  spline S106 degree 2 poles (-1.5969, 23.0765) (-1.2112, 23.0765) (-0.7744, 22.566) (-0.7744, 22.081) knots 0 0 0 1 2 2 2
  line L155 (-0.7744, 22.081) -> (-0.7744, 20.3763)
  spline S107 degree 2 poles (0.6409, 20.3253) (0.2807, 20.3253) (-0.1249, 20.7366) (-0.1249, 21.1819) knots 0 0 0 1 2 2 2
  line L156 (-0.1249, 21.1819) -> (-0.1249, 22.6369)
  line L157 (-0.1249, 22.6369) -> (-0.4227, 22.6369)
  line L158 (-0.4227, 22.6369) -> (-0.4227, 23.0028)
  line L159 (-0.4227, 23.0028) -> (-0.1249, 23.0028)
  line L160 (-0.1249, 23.0028) -> (-0.1249, 23.7572)
  line L161 (-0.1249, 23.7572) -> (0.3176, 23.7572)
  line L162 (0.3176, 23.7572) -> (0.3176, 23.0028)
  line L163 (0.3176, 23.0028) -> (1.1316, 23.0028)
  line L164 (1.1316, 23.0028) -> (1.1316, 22.6369)
  line L165 (1.1316, 22.6369) -> (0.3176, 22.6369)
  line L166 (0.3176, 22.6369) -> (0.3176, 21.3861)
  spline S108 degree 2 poles (0.3176, 21.3861) (0.3176, 21.1875) (0.3318, 20.9691) (0.38, 20.8755) knots 0 0 0 1 2 2 2
  spline S109 degree 2 poles (0.38, 20.8755) (0.4197, 20.7933) (0.5984, 20.711) (0.7515, 20.711) knots 0 0 0 1 2 2 2
  spline S110 degree 2 poles (0.7515, 20.711) (0.8593, 20.711) (1.0607, 20.7763) (1.1061, 20.7961) knots 0 0 0 1 2 2 2
  line L167 (1.1061, 20.7961) -> (1.1316, 20.7961)
  line L168 (1.1316, 20.7961) -> (1.1316, 20.399)
  spline S111 degree 2 poles (1.1316, 20.399) (1.0068, 20.365) (0.7515, 20.3253) (0.6409, 20.3253) knots 0 0 0 1 2 2 2
  spline S112 degree 2 poles (2.598, 20.3168) (1.9683, 20.3168) (1.2763, 21.023) (1.2763, 21.6754) knots 0 0 0 1 2 2 2
  spline S113 degree 2 poles (1.2763, 21.6754) (1.2763, 22.3164) (1.9485, 23.0765) (2.4902, 23.0765) knots 0 0 0 1 2 2 2
  spline S114 degree 2 poles (2.4902, 23.0765) (2.7341, 23.0765) (3.1113, 22.9347) (3.2503, 22.7844) knots 0 0 0 1 2 2 2
  spline S115 degree 2 poles (3.2503, 22.7844) (3.3921, 22.634) (3.5425, 22.2001) (3.5425, 21.8853) knots 0 0 0 1 2 2 2
  line L169 (3.5425, 21.8853) -> (3.5425, 21.6442)
  line L170 (3.5425, 21.6442) -> (1.7244, 21.6442)
  spline S116 degree 2 poles (1.7244, 21.6442) (1.7244, 21.1875) (2.1839, 20.7025) (2.5923, 20.7025) knots 0 0 0 1 2 2 2
  spline S117 degree 2 poles (2.5923, 20.7025) (2.737, 20.7025) (3.0178, 20.7678) (3.1312, 20.8188) knots 0 0 0 1 2 2 2
  spline S118 degree 2 poles (3.1312, 20.8188) (3.2503, 20.8755) (3.4148, 20.9748) (3.4687, 21.0202) knots 0 0 0 1 2 2 2
  line L171 (3.4687, 21.0202) -> (3.4943, 21.0202)
  line L172 (3.4943, 21.0202) -> (3.4943, 20.538)
  spline S119 degree 2 poles (3.4943, 20.538) (3.4177, 20.5068) (3.1851, 20.4161) (3.0943, 20.3905) knots 0 0 0 1 2 2 2
  spline S120 degree 2 poles (3.0943, 20.3905) (2.9667, 20.3537) (2.7568, 20.3168) (2.598, 20.3168) knots 0 0 0 1 2 2 2
  spline S121 degree 2 poles (3.1113, 21.9817) (3.1057, 22.1604) (3.0319, 22.4213) (2.961, 22.5092) knots 0 0 0 1 2 2 2
  spline S122 degree 2 poles (2.961, 22.5092) (2.8844, 22.6085) (2.6434, 22.7135) (2.4647, 22.7135) knots 0 0 0 1 2 2 2
  spline S123 degree 2 poles (2.4647, 22.7135) (2.2888, 22.7135) (2.0421, 22.6085) (1.94, 22.5064) knots 0 0 0 1 2 2 2
  spline S124 degree 2 poles (1.94, 22.5064) (1.8407, 22.4015) (1.7386, 22.149) (1.7244, 21.9817) knots 0 0 0 1 2 2 2
  line L173 (1.7244, 21.9817) -> (3.1113, 21.9817)
  line L174 (4.4416, 20.3763) -> (3.9991, 20.3763)
  line L175 (3.9991, 20.3763) -> (3.9991, 23.0028)
  line L176 (3.9991, 23.0028) -> (4.4416, 23.0028)
  line L177 (4.4416, 23.0028) -> (4.4416, 20.3763)
  line L178 (4.4728, 23.4396) -> (3.9707, 23.4396)
  line L179 (3.9707, 23.4396) -> (3.9707, 23.899)
  line L180 (3.9707, 23.899) -> (4.4728, 23.899)
  line L181 (4.4728, 23.899) -> (4.4728, 23.4396)
  line L182 (6.4837, 22.5291) -> (6.461, 22.5291)
  spline S125 degree 2 poles (6.461, 22.5291) (6.41, 22.5433) (6.2994, 22.549) (6.2228, 22.549) knots 0 0 0 1 2 2 2
  spline S126 degree 2 poles (6.2228, 22.549) (6.0441, 22.549) (5.6924, 22.393) (5.5336, 22.2398) knots 0 0 0 1 2 2 2
  line L183 (5.5336, 22.2398) -> (5.5336, 20.3763)
  line L184 (5.5336, 20.3763) -> (5.0911, 20.3763)
  line L185 (5.0911, 20.3763) -> (5.0911, 23.0028)
  line L186 (5.0911, 23.0028) -> (5.5336, 23.0028)
  line L187 (5.5336, 23.0028) -> (5.5336, 22.6114)
  spline S127 degree 2 poles (5.5336, 22.6114) (5.7746, 22.8269) (6.1348, 23.0028) (6.305, 23.0028) knots 0 0 0 1 2 2 2
  spline S128 degree 2 poles (6.305, 23.0028) (6.3731, 23.0028) (6.4412, 22.9971) (6.4837, 22.9886) knots 0 0 0 1 2 2 2
  line L188 (6.4837, 22.9886) -> (6.4837, 22.5291)
  spline S129 degree 2 poles (8.9853, 21.6896) (8.9853, 21.0259) (8.3472, 20.3026) (7.8139, 20.3026) knots 0 0 0 1 2 2 2
  spline S130 degree 2 poles (7.8139, 20.3026) (7.2665, 20.3026) (6.6397, 21.0486) (6.6397, 21.6896) knots 0 0 0 1 2 2 2
  spline S131 degree 2 poles (6.6397, 21.6896) (6.6397, 22.3476) (7.2864, 23.0765) (7.8139, 23.0765) knots 0 0 0 1 2 2 2
  spline S132 degree 2 poles (7.8139, 23.0765) (8.3472, 23.0765) (8.9853, 22.3504) (8.9853, 21.6896) knots 0 0 0 1 2 2 2
  spline S133 degree 2 poles (8.5287, 21.6896) (8.5287, 22.2001) (8.1571, 22.6964) (7.8139, 22.6964) knots 0 0 0 1 2 2 2
  spline S134 degree 2 poles (7.8139, 22.6964) (7.4707, 22.6964) (7.0964, 22.2001) (7.0964, 21.6896) knots 0 0 0 1 2 2 2
  spline S135 degree 2 poles (7.0964, 21.6896) (7.0964, 21.1932) (7.4707, 20.6827) (7.8139, 20.6827) knots 0 0 0 1 2 2 2
  spline S136 degree 2 poles (7.8139, 20.6827) (8.1543, 20.6827) (8.5287, 21.1847) (8.5287, 21.6896) knots 0 0 0 1 2 2 2
  line L189 (-16.7357, 14.6137) -> (-15.5558, 18.1137)
  line L190 (-15.5558, 18.1137) -> (-14.9829, 18.1137)
  line L191 (-14.9829, 18.1137) -> (-13.803, 14.6137)
  line L192 (-13.803, 14.6137) -> (-14.2936, 14.6137)
  line L193 (-14.2936, 14.6137) -> (-14.6113, 15.5922)
  line L194 (-14.6113, 15.5922) -> (-15.9472, 15.5922)
  line L195 (-15.9472, 15.5922) -> (-16.2649, 14.6137)
  line L196 (-16.2649, 14.6137) -> (-16.7357, 14.6137)
  line L197 (-14.7389, 15.9893) -> (-15.2807, 17.6372)
  line L198 (-15.2807, 17.6372) -> (-15.8196, 15.9893)
  line L199 (-15.8196, 15.9893) -> (-14.7389, 15.9893)
  line L200 (-13.8483, 14.6137) -> (-12.6684, 18.1137)
  line L201 (-12.6684, 18.1137) -> (-12.0955, 18.1137)
  line L202 (-12.0955, 18.1137) -> (-10.9156, 14.6137)
  line L203 (-10.9156, 14.6137) -> (-11.4063, 14.6137)
  line L204 (-11.4063, 14.6137) -> (-11.7239, 15.5922)
  line L205 (-11.7239, 15.5922) -> (-13.0598, 15.5922)
  line L206 (-13.0598, 15.5922) -> (-13.3775, 14.6137)
  line L207 (-13.3775, 14.6137) -> (-13.8483, 14.6137)
  line L208 (-11.8516, 15.9893) -> (-12.3933, 17.6372)
  line L209 (-12.3933, 17.6372) -> (-12.9322, 15.9893)
  line L210 (-12.9322, 15.9893) -> (-11.8516, 15.9893)
  line L211 (-8.5246, 14.6137) -> (-10.683, 14.6137)
  line L212 (-10.683, 14.6137) -> (-10.683, 15.11)
  spline S137 degree 2 poles (-10.683, 15.11) (-10.4504, 15.3284) (-10.0363, 15.734) (-9.8378, 15.9524) knots 0 0 0 1 2 2 2
  spline S138 degree 2 poles (-9.8378, 15.9524) (-9.4379, 16.3921) (-9.1457, 16.9196) (-9.1457, 17.2004) knots 0 0 0 1 2 2 2
  spline S139 degree 2 poles (-9.1457, 17.2004) (-9.1457, 17.3479) (-9.2365, 17.5691) (-9.3188, 17.64) knots 0 0 0 1 2 2 2
  spline S140 degree 2 poles (-9.3188, 17.64) (-9.401, 17.7109) (-9.6166, 17.7818) (-9.747, 17.7818) knots 0 0 0 1 2 2 2
  spline S141 degree 2 poles (-9.747, 17.7818) (-9.8718, 17.7818) (-10.1271, 17.7194) (-10.2434, 17.6712) knots 0 0 0 1 2 2 2
  spline S142 degree 2 poles (-10.2434, 17.6712) (-10.3427, 17.6315) (-10.527, 17.5181) (-10.5837, 17.4784) knots 0 0 0 1 2 2 2
  line L213 (-10.5837, 17.4784) -> (-10.6093, 17.4784)
  line L214 (-10.6093, 17.4784) -> (-10.6093, 17.9775)
  spline S143 degree 2 poles (-10.6093, 17.9775) (-10.4646, 18.0485) (-9.9456, 18.1874) (-9.713, 18.1874) knots 0 0 0 1 2 2 2
  spline S144 degree 2 poles (-9.713, 18.1874) (-9.2223, 18.1874) (-8.6692, 17.6684) (-8.6692, 17.2259) knots 0 0 0 1 2 2 2
  spline S145 degree 2 poles (-8.6692, 17.2259) (-8.6692, 17.0189) (-8.7657, 16.6728) (-8.8508, 16.5254) knots 0 0 0 1 2 2 2
  spline S146 degree 2 poles (-8.8508, 16.5254) (-8.9359, 16.3722) (-9.1826, 16.0715) (-9.3188, 15.9269) knots 0 0 0 1 2 2 2
  spline S147 degree 2 poles (-9.3188, 15.9269) (-9.54, 15.6858) (-10.0817, 15.1696) (-10.2434, 15.0193) knots 0 0 0 1 2 2 2
  line L215 (-10.2434, 15.0193) -> (-8.5246, 15.0193)
  line L216 (-8.5246, 15.0193) -> (-8.5246, 14.6137)
  line L217 (-7.1405, 14.6137) -> (-7.1405, 17.6996)
  line L218 (-7.1405, 17.6996) -> (-8.3147, 17.6996)
  line L219 (-8.3147, 17.6996) -> (-8.3147, 18.1137)
  line L220 (-8.3147, 18.1137) -> (-5.5011, 18.1137)
  line L221 (-5.5011, 18.1137) -> (-5.5011, 17.6996)
  line L222 (-5.5011, 17.6996) -> (-6.6753, 17.6996)
  line L223 (-6.6753, 17.6996) -> (-6.6753, 14.6137)
  line L224 (-6.6753, 14.6137) -> (-7.1405, 14.6137)
  line L225 (-2.7272, 14.6137) -> (-3.2604, 14.6137)
  line L226 (-3.2604, 14.6137) -> (-4.1113, 16.0092)
  line L227 (-4.1113, 16.0092) -> (-4.9792, 14.6137)
  line L228 (-4.9792, 14.6137) -> (-5.4812, 14.6137)
  line L229 (-5.4812, 14.6137) -> (-4.3666, 16.3665)
  line L230 (-4.3666, 16.3665) -> (-5.4472, 18.1137)
  line L231 (-5.4472, 18.1137) -> (-4.914, 18.1137)
  line L232 (-4.914, 18.1137) -> (-4.0801, 16.7438)
  line L233 (-4.0801, 16.7438) -> (-3.2292, 18.1137)
  line L234 (-3.2292, 18.1137) -> (-2.7272, 18.1137)
  line L235 (-2.7272, 18.1137) -> (-3.822, 16.3892)
  line L236 (-3.822, 16.3892) -> (-2.7272, 14.6137)
  point P0 (0, 0)
  constraints: 2 other
emboss "Emboss1" sketch "Sketch13" operation cut depth 0.1 direction (0, 0, -1)
equation "\"d19\" = BendReliefWidth"
equation "\"d20\" = BendReliefDepth"
equation "\"d21\" = MinimumRemnant"
equation "\"d22\" = BendRadius"
equation "\"d24\" = BendRadius"
equation "\"d26\" = BendReliefWidth"
equation "\"d27\" = BendReliefDepth"
equation "\"d28\" = MinimumRemnant"
equation "\"d29\" = BendRadius"
equation "\"d31\" = BendRadius"
equation "\"d33\" = BendReliefWidth"
equation "\"d34\" = BendReliefDepth"
equation "\"d35\" = MinimumRemnant"
equation "\"d36\" = BendRadius"
equation "\"d38\" = BendRadius"
equation "\"d40\" = BendReliefWidth"
equation "\"d41\" = BendReliefDepth"
equation "\"d42\" = MinimumRemnant"
equation "\"d43\" = BendRadius"
equation "\"d45\" = BendRadius"
equation "\"d47\" = BendReliefWidth"
equation "\"d48\" = BendReliefDepth"
equation "\"d49\" = MinimumRemnant"
equation "\"d50\" = BendRadius"
equation "\"d52\" = BendRadius"
equation "\"d54\" = BendReliefWidth"
equation "\"d55\" = BendReliefDepth"
equation "\"d56\" = MinimumRemnant"
equation "\"d57\" = BendRadius"
equation "\"d59\" = BendRadius"
equation "\"BendReliefWidth\" = Thickness"
equation "\"BendReliefDepth\" = 0.5 * Thickness"
equation "\"CornerReliefSize\" = 4 * Thickness"
equation "\"MinimumRemnant\" = 2 * Thickness"
equation "\"TransitionRadius\" = BendRadius"
equation "\"JacobiRadiusSize\" = BendRadius"
equation "\"GapSize\" = Thickness"
equation "\"d11\" = BendRadius"
equation "\"BendRadius\" = 0.001"
equation "\"Thickness\" = 0.381"
body "Solid1"
